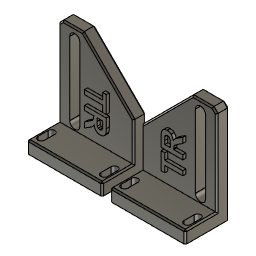
Y#motor_holder_extrusion R+L (Autodesk Fusion 360 design; units mm, degrees)
Autodesk Fusion 360 part; units mm, degrees
note: some values were not read from the file. Set by a fixed rule: which face or edge a step refers to.
sketch "Sketch1" plane through (0, 0, 0) normal (0, 0, 1) x (1, 0, 0)
  circle A0 centre (0, 0) radius 1.65
  line L0 (0, 0) -> (31, 0)
  circle A1 centre (31, 0) radius 1.65
  line L1 (1.65, 0) -> (1.65, 11.5)
  line L2 (1.65, 11.5) -> (1.65, 17.5)
  line L3 (1.65, 17.5) -> (51.65, 17.5)
  line L4 (31, 0) -> (26, 0)
  line L5 (26, 0) -> (26, 17.5)
  line L6 (0, 0) -> (-3, -4)
  line L7 (31, 0) -> (34, -4)
  line L8 (34, -4) -> (-3, -4)
  line L9 (-3, -4) -> (-3, 17.5)
  line L10 (-3, 17.5) -> (1.65, 17.5)
  line L11 (34, -4) -> (34, 17.5)
  line L12 (-3, 17.5) -> (47, 17.5)
  line L13 (47, 17.5) -> (47, 11.5)
  line L14 (47, 11.5) -> (-3, 11.5)
  line L15 (-3, 11.5) -> (-3, 17.5)
  dimension "d1" = 3.3
  dimension "d2" = 31
  dimension "d3" = 3.3
  dimension "d4" = 11.5
  dimension "d5" = 6
  dimension "d6" = 50
  dimension "d7" = 50
  dimension "d8" = 6
  constraint coincident A0.centre L0.start
  constraint horizontal L0
  constraint coincident L0.end A1.centre
  constraint coincident A0 L1.start
  constraint coincident L0 L1.start
  constraint perpendicular L0 L1
  constraint parallel L1 L2
  constraint perpendicular L2 L3
  constraint coincident L0 L4.end
  constraint coincident L3 L5.end
  constraint perpendicular L3 L5
  constraint horizontal L8
  constraint perpendicular L3 L9
  constraint perpendicular L2 L10
  constraint coincident L3 L11.end
  constraint perpendicular L3 L11
  constraint horizontal L12
  constraint vertical L13
  constraint horizontal L14
  constraint vertical L15
  measures "d1" diameter of A0
  measures "d2" distance of A0.centre L0.end
  measures "d3" diameter of A1
  measures "d4" distance of L1.start L1.end
  measures "d5" distance of L1.end L2.end
  measures "d6" distance of L2.end L3.end
  measures "d7" distance of L9.end L12.end
  measures "d8" distance of L9.end L14.end
extrude "Extrude1" add sketch "Sketch1" along normal blind 30 contours L2 L9 L10 L12 L14 L15 | L2 L3 L5 L12 L14 | L3 L5 L11 L12 L14 | L3 L11 L12 L13 L14 makes body 1
extrude "Extrude2" add sketch "Sketch1" along normal blind 6 contours A0 L0 A1 L4 L6 L7 L8 | L0 L1 L5 L14 | A0 L1 L6 L9 L14 | L0 A1 L4 L5 L7 L11 L14 bodies 1
extrude "Extrude3" cut 1 faces at (47, 15.5, 10) along direction (-1, 0, 0) blind 13 on bodies 1 bodies 1
extrude "Extrude4" add 1 faces at (21.6667, 13.5, 30) along direction (0, 0, 1) blind 20 on bodies 1 bodies 1
sketch "Sketch2" plane through (0, 11.5, 0) normal (0, -1, 0) x (1, 0, 0)
  line L0 (34, 6) -> (34, 50)
  line L1 (34, 50) -> (-3, 50)
  line L2 (-3, 50) -> (-3, 6)
  line L3 (-3, 6) -> (34, 6)
  line L4 (34, 6) -> (26, 6)
  line L5 (28.5, 9) -> (28.5, 45)
  arc A0 (28.5, 45) -> (23.5, 45) centre (26, 45) ccw
  line L6 (23.5, 45) -> (23.5, 9)
  arc A1 (23.5, 9) -> (28.5, 9) centre (26, 9) ccw
  line L7 (26, 9) -> (26, 45) construction
  dimension "d17" = 5
  constraint coincident L0.start L3.end
  constraint coincident L3 L4.end
  constraint parallel L3 L4
  constraint tangent L5 A0
  constraint tangent A0 L6
  constraint parallel L5 L6
  constraint tangent L6 A1
  constraint tangent L5 A1
  measures "d17" diameter of A0
extrude "Extrude5" cut sketch "Sketch2" against normal blind 56 contours L5 A0 L6 A1 bodies 1
chamfer "Chamfer1" distance 25 angle 45 1 edges at (-3, 14.5, 50) on bodies 1
chamfer "Chamfer2" distance 2 angle 45 1 edges at (34, 14.5, 50) on bodies 1
chamfer "Chamfer3" distance 0.7 angle 45 15 edges at (-3, 17.5, 12.5) (9.5, 17.5, 37.5) (27, 17.5, 50) (33, 17.5, 49) (34, 17.5, 24) (-3, -4, 3) (-3, 3.75, 6) (-3, 11.5, 15.5) (9.5, 11.5, 37.5) (27, 11.5, 50) (15.5, -4, 6) (34, -4, 3) (34, 3.75, 6) (34, 11.5, 27) (33, 11.5, 49) on bodies 1
sketch "Sketch3" plane through (0, 0, 6) normal (0, 0, 1) x (-1, 0, 0)
  line L0 (2.3, -11.5) -> (2.3, 3.3)
  line L1 (2.3, 3.3) -> (-33.3, 3.3)
  line L2 (-33.3, 3.3) -> (-33.3, -11.5)
  line L3 (-33.3, -11.5) -> (2.3, -11.5)
  circle A0 centre (0, 0) radius 1.65
  circle A1 centre (-31, 0) radius 1.65
  line L4 (-1.65, 0) -> (-1.65, -5)
  arc A2 (-1.65, -5) -> (1.65, -5) centre (0, -5) ccw
  line L5 (1.65, -5) -> (1.65, 0)
  arc A3 (1.65, 0) -> (-1.65, 0) centre (0, 0) ccw
  line L6 (0, 0) -> (0, -5) construction
  line L7 (-32.65, 0) -> (-32.65, -5)
  arc A4 (-32.65, -5) -> (-29.35, -5) centre (-31, -5) ccw
  line L8 (-29.35, -5) -> (-29.35, 0)
  arc A5 (-29.35, 0) -> (-32.65, 0) centre (-31, 0) ccw
  line L9 (-31, 0) -> (-31, -5) construction
  dimension "d23" = 3.3
  dimension "d24" = 3.3
  constraint tangent L4 A2
  constraint tangent A2 L5
  constraint parallel L4 L5
  constraint tangent L5 A3
  constraint tangent L4 A3
  constraint perpendicular L1 L6
  constraint coincident A0.centre A3.centre
  constraint tangent L7 A4
  constraint tangent A4 L8
  constraint parallel L7 L8
  constraint tangent L8 A5
  constraint tangent L7 A5
  constraint perpendicular L1 L9
  constraint coincident A1.centre A5.centre
  measures "d23" diameter of A2
  measures "d24" diameter of A4
extrude "Extrude6" cut sketch "Sketch3" against normal blind 5 contours A0 L4 A2 L5 | A1 L7 A4 L8 bodies 1
extrude "Extrude7" cut 2 faces at (-0.0411, 3.8818, 1) (30.9589, 3.8818, 1) along direction (0, 0, -1) blind 50 on bodies 1 bodies 1
sketch "Sketch4" plane through (0, 11.5, 0) normal (0, -1, 0) x (1, 0, 0)
  line L0 (-2.3, 24.7101) -> (-2.3, 6)
  line L1 (-2.3, 6) -> (33.3, 6)
  line L2 (33.3, 6) -> (33.3, 47.7101)
  line L3 (33.3, 47.7101) -> (31.7101, 49.3)
  line L4 (31.7101, 49.3) -> (22.2899, 49.3)
  line L5 (22.2899, 49.3) -> (-2.3, 24.7101)
  line L6 (28.5, 45) -> (28.5, 9)
  arc A0 (23.5, 9) -> (28.5, 9) centre (26, 9) ccw
  line L7 (23.5, 9) -> (23.5, 45)
  arc A1 (28.5, 45) -> (23.5, 45) centre (26, 45) ccw
  line L8 (18.8103, 11.6668) -> (18.8103, 31.2152) construction
  line L9 (18.8103, 31.2152) -> (3.8103, 31.2152) construction
  line L10 (3.8103, 31.2152) -> (3.8103, 11.6668) construction
  line L11 (3.8103, 11.6668) -> (18.8103, 11.6668) construction
  text T0 "TR" font "Arial" height 15 bold align ink ink in box 0 x 0 at (18.7903, 11.6768) x (0, 1) y (-1, 0) spacing 1 height is em
  constraint perpendicular L8 L9
  constraint parallel L8 L10
  constraint parallel L9 L11
extrude "Extrude8" add sketch "Sketch4" along normal blind 1 text T0 bodies 1
extrude "Extrude9" add 2 faces at (12.843, 10.5, 16.3082) (13.1457, 10.5, 22.3385) along direction (0, -1, 0) blind 0.5 on bodies 1 bodies 1
mirror "Mirror1" about plane through (0, 0, 0) normal (1, 0, 0) of bodies 1 makes body 2
move_body "Move1" bodies 2 to x (1, 0, 0) y (0, 1, 0) z (0, 0, 1) at (-10, 0, 0)
extrude "Extrude10" cut 2 faces at (-22.843, 10, 16.3082) (-23.1457, 10, 22.3385) along direction (0, 1, 0) blind 1 on bodies 2 bodies 2
extrude "Extrude11" cut 2 faces at (-22.843, 11, 16.3082) (-23.1457, 11, 22.3385) along direction (0, 1, 0) blind 0.5 on bodies 2 bodies 2
sketch "Sketch5" plane through (0, 11.5, 0) normal (0, -1, 0) x (1, 0, 0)
  line L0 (-7.7, 6) -> (-7.7, 24.7101)
  line L1 (-7.7, 24.7101) -> (-32.2899, 49.3)
  line L2 (-32.2899, 49.3) -> (-41.7101, 49.3)
  line L3 (-41.7101, 49.3) -> (-43.3, 47.7101)
  line L4 (-43.3, 47.7101) -> (-43.3, 6)
  line L5 (-43.3, 6) -> (-7.7, 6)
  line L6 (-38.5, 9) -> (-38.5, 45)
  arc A0 (-33.5, 45) -> (-38.5, 45) centre (-36, 45) ccw
  line L7 (-33.5, 45) -> (-33.5, 9)
  arc A1 (-38.5, 9) -> (-33.5, 9) centre (-36, 9) ccw
  line L8 (-29.7239, 30.6211) -> (-29.7239, 11.0728) construction
  line L9 (-29.7239, 11.0728) -> (-14.7239, 11.0728) construction
  line L10 (-14.7239, 11.0728) -> (-14.7239, 30.6211) construction
  line L11 (-14.7239, 30.6211) -> (-29.7239, 30.6211) construction
  text T0 "TR" font "Arial" height 15 bold align ink ink in box 0 x 0 at (-29.7039, 30.6111) x (0, -1) y (1, 0) spacing 1 height is em
  constraint perpendicular L8 L9
  constraint parallel L8 L10
  constraint parallel L9 L11
extrude "Extrude12" add sketch "Sketch5" along normal blind 1.5 text T0 bodies 2
